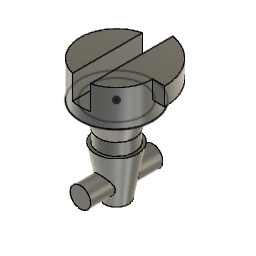
Fluke 87-V Battery Screw (Autodesk Fusion 360 design; units mm, degrees)
Autodesk Fusion 360 part; units mm, degrees
note: some values were not read from the file. Set by a fixed rule: which sketch regions a step uses.
sketch "Sketch1" plane through (0, 0, 0) normal (0, 0, 1) x (1, 0, 0) in component "Battery Screw"
  circle A0 centre (0, 0) radius 3.81
  circle A1 centre (0, 0) radius 2.8575
  dimension "d3" = 7.62
  dimension "d14" = 5.715
  constraint coincident A0.centre A1.centre
  measures "d3" diameter of A0
  measures "d14" diameter of A1
extrude "Extrude2" add sketch "Sketch1" along normal blind 3.81 contours A0 | A1 in component "Battery Screw"
sketch "Sketch2" plane through (0, 0, 3.81) normal (0, 0, 1) x (-1, 0, 0) in component "Battery Screw"
  circle A0 centre (0, 0) radius 3.81
  line L0 (-0.9525, -6.35) -> (0.9525, -6.35)
  line L1 (0.9525, -6.35) -> (0.9525, 6.35)
  line L2 (0.9525, 6.35) -> (-0.9525, 6.35)
  line L3 (-0.9525, 6.35) -> (-0.9525, -6.35)
  line L4 (-0.9525, -6.35) -> (0.9525, 6.35) construction
  line L5 (0.9525, -6.35) -> (-0.9525, 6.35) construction
  dimension "d6" = 1.905
  dimension "d7" = 12.7
  constraint horizontal L0
  constraint perpendicular L0 L1
  constraint parallel L0 L2
  constraint parallel L1 L3
  constraint coincident L4 A0.centre
  constraint coincident L5 A0.centre
  constraint coincident A0.centre origin
  measures "d6" distance of L1.end L2.end
  measures "d7" distance of L0.end L1.end
extrude "Extrude3" cut sketch "Sketch2" against normal blind 2.54 contours A0 L1 L3 | A0 L1 L2 L3 | A0 L0 L1 L3 in component "Battery Screw"
sketch "Sketch3" plane through (0, 0, 3.81) normal (0, 0, 1) x (-1, 0, 0) in component "Battery Screw"
  arc A0 (-0.9525, 3.689) -> (-0.9525, -3.689) centre (0, 0) ccw
  line L0 (0, 0) -> (0, -5.08)
  line L1 (0, 0) -> (-5.08, 0)
  arc A1 (-5.08, 0) -> (0, -5.08) centre (0, 0) ccw
  circle A2 centre (0, 0) radius 3.81
  line L2 (-0.9525, -3.689) -> (-0.9525, 3.689)
  line L3 (0.9525, 3.689) -> (0.9525, -3.689)
  arc A3 (0.9525, -3.689) -> (0.9525, 3.689) centre (0, 0) ccw
  line L4 (-0.9525, 0) -> (-0.9525, -4.9899)
  dimension "d11" = 1.27
  constraint coincident A0.centre L0.start
  constraint perpendicular L0 L1
  constraint parallel L0 L2
  constraint midpoint L2 L4.start
  constraint coincident A1 L4.end
  constraint parallel L2 L4
  measures "d11" distance of A1 A2
extrude "Extrude4" add sketch "Sketch3" against normal blind 1.905 contours A0 L1 A1 A2 L4 in component "Battery Screw"
ref_plane "WorkPlane1" through (0, 0, -2.54) normal (0, 0, 1) x (1, 0, 0) in component "Battery Screw"
sketch "Sketch4" plane through (0, 0, -2.54) normal (0, 0, 1) x (1, 0, 0) in component "Battery Screw"
  circle A0 centre (0, 0) radius 1.905
  dimension "d16" = 3.81
  constraint coincident A0.centre origin
  measures "d16" diameter of A0
loft "Loft1" add profiles "Sketch1", "Sketch4" section 1 contours A1 section 2 in component "Battery Screw"
extrude "Extrude5" add 1 faces at (-0.3367, 0.2932, -2.54) along direction (0, 0, -1) blind 1.27 in component "Battery Screw"
sketch "Sketch5" plane through (0, 0, -3.81) normal (0, 0, -1) x (1, 0, 0) in component "Battery Screw"
  circle A0 centre (0, 0) radius 1.905
  circle A1 centre (0, 0) radius 2.2225
  dimension "d19" = 4.445
  constraint concentric A0 A1
  measures "d19" diameter of A1
ref_plane "WorkPlane2" through (0, 0, -8.89) normal (0, 0, -1) x (1, 0, 0) in component "Battery Screw"
sketch "Sketch6" plane through (0, 0, -8.89) normal (0, 0, -1) x (1, 0, 0) in component "Battery Screw"
sketch "Sketch7" plane through (0, 0, -8.89) normal (0, 0, -1) x (1, 0, 0) in component "Battery Screw"
  circle A0 centre (0, 0) radius 1.27
  dimension "d21" = 2.54
  constraint coincident A0.centre origin
  measures "d21" diameter of A0
loft "Loft2" add profiles "Sketch5", "Sketch7" section 1 contours A0 | A1 section 2 in component "Battery Screw"
ref_plane "WorkPlane3" through (0, -3.81, 1.0847) normal (0, -1, 0) x (-1, 0, 0) in component "Battery Screw"
sketch "Sketch8" plane through (0, -3.81, 1.0847) normal (0, -1, 0) x (1, 0, 0) in component "Battery Screw"
  line L0 (-2.2225, -4.8947) -> (2.2225, -4.8947)
  line L1 (1.27, -9.9747) -> (-1.27, -9.9747)
  line L2 (0, -9.9747) -> (0, -8.0697)
  circle A0 centre (0, -8.0697) radius 1.0795
  dimension "d23" = 1.905
  dimension "d24" = 2.159
  constraint midpoint L1 L2.start
  constraint perpendicular L1 L2
  constraint coincident L2.end A0.centre
  measures "d23" distance of L2.start L2.end
  measures "d24" diameter of A0
extrude "Extrude6" add sketch "Sketch8" against normal blind 7.62 in component "Battery Screw"
component "Battery Screw" placed x (1, 0, 0) y (0, 1, 0) z (0, 0, 1) at (0, 0, 0)
equation "d23 = 0.05 in + 0.025 in"
